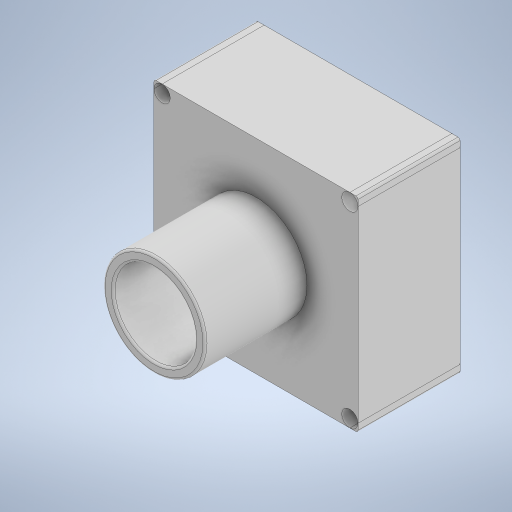
# Autodesk Inventor part: Práctica 1
Saved by Autodesk Inventor 2024 (Build 280153000, 153)
## iProperties
Created: 2024-02-19
Part Number: Práctica 1
Material: Generic
Document SubType Name: Modeling
Designer: sebas
Density: 1 g/cm^3
Appearance: Default
Author: sebas
Autodesk Inventor part; units mm, degrees
ref_plane "YZ Plane" through (0, 0, 0) normal (1, 0, 0) x (0, 1, 0)
ref_plane "XZ Plane" through (0, 0, 0) normal (0, 1, 0) x (-1, 0, 0)
ref_plane "XY Plane" through (0, 0, 0) normal (0, 0, 1) x (1, 0, 0)
sketch "Sketch1" plane through (0, 0, 0) normal (0, 0, 1) x (1, 0, 0)
  line L0 (0, 0) -> (1000, 0)
  line L1 (1000, 0) -> (1000, -1000)
  line L2 (1000, -1000) -> (0, -1000)
  line L3 (0, -1000) -> (0, 0)
  dimension "d0" = 1000
  dimension "d1" = 1000
  constraints: 8 end point, 2 parallel, 1 coincident, 1 horizontal, 1 perpendicular
  measures "d0" distance of L1.end L2.end
  measures "d1" distance of L0.end L1.end
extrude "Extrusion1" add sketch "Sketch1" along normal blind 500
sketch "Sketch2" plane through (0, 0, 500) normal (0, 0, 1) x (1, 0, 0)
  line L0 (0, 0) -> (0, -1000) projected
  line L1 (0, -500) -> (1000, -500) construction
  line L2 (1000, -1000) -> (1000, 0) projected
  circle A0 centre (500, -500) radius 250
  dimension "d4" = 500
  constraints: 3 midpoint, 2 end point, 1 centre point
  measures "d4" diameter of A0
extrude "Extrusion2" add sketch "Sketch2" along normal blind 500
sketch "Sketch3" plane through (500, -500, 1000) normal (0, 0, 1) x (1, 0, 0)
  circle A0 centre (0, 0) radius 250 projected
  circle A1 centre (0, 0) radius 200
  point P0 (-500, 500)
  dimension "d7" = 400
  constraints: 1 centre point, 1 coincident
  measures "d7" diameter of A1
extrude "Extrusion3" cut sketch "Sketch3" against normal blind 300 contours A1
fillet "Fillet1" radius 10 5 edges at (1000, 0, 250) (1000, -1000, 250) (0, 0, 250) (0, -1000, 250) (300, -500, 1000)
sketch "Sketch4" plane through (0, 0, 500) normal (0, 0, 1) x (1, 0, 0)
  line L0 (0, -10) -> (0, -990) projected
  line L1 (1000, -990) -> (1000, -10) projected
  line L2 (10, -1000) -> (990, -1000) projected
  line L3 (-34.7433, -960) -> (1071.285, -960) construction
  line L4 (960, -1052.4238) -> (960, 91.4593) construction
  line L5 (990, 0) -> (10, 0) projected
  circle A0 centre (960, -960) radius 40
  line L6 (1056.705, -40) -> (-70.4177, -40) construction
  line L7 (40, 72.2034) -> (40, -1093.9026) construction
  circle A1 centre (40, -960) radius 40
  circle A2 centre (40, -40) radius 40
  circle A3 centre (960, -40) radius 40
  point P0 (0, 0)
  point P1 (960, -1052.4238)
  point P2 (960, 91.4593)
  dimension "d12" = 40
  dimension "d13" = 40
  dimension "d14" = 80
  dimension "d15" = 40
  dimension "d16" = 40
  dimension "d17" = 80
  dimension "d18" = 80
  dimension "d19" = 80
  constraints: 6 end point, 6 point on line, 4 centre point, 2 horizontal, 1 perpendicular, 1 vertical, 5 other
  measures "d12" distance between parallel lines of L2 L3
  measures "d14" diameter of A0
  measures "d15" distance between parallel lines of L5 L6
  measures "d16" distance between parallel lines of L7 L0
  measures "d17" diameter of A1
  measures "d18" diameter of A2
  measures "d19" diameter of A3
extrude "Extrusion4" cut sketch "Sketch4" against normal blind 500 contours A2 | A1 | A3 | A0
fillet "Fillet2" radius 10 1 edges at (250, -500, 1000)
body "Solid1"
